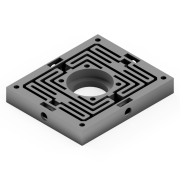
# Autodesk Inventor part: PinholeFlexMain
Saved by Autodesk Inventor 2022 (Build 260153000, 153)
## iProperties
Created: 2022-05-14
Part Number: PinholeFlexMain
Material: Acetal Resin, Black
Document SubType Name: Modeling
Designer: eganc
Density: 1.425 g/cm^3
Appearance: Smooth - Black
Author: eganc
Autodesk Inventor part; units mm, degrees
ref_plane "YZ Plane" through (0, 0, 0) normal (1, 0, 0) x (0, 1, 0)
ref_plane "XZ Plane" through (0, 0, 0) normal (0, 1, 0) x (-1, 0, 0)
ref_plane "XY Plane" through (0, 0, 0) normal (0, 0, 1) x (1, 0, 0)
sketch "Sketch1" plane through (0, 0, 0) normal (0, 1, 0) x (-1, 0, 0)
  line L0 (-14.5, 17.5) -> (14.5, 17.5)
  line L1 (14.5, 17.5) -> (14.5, -17.5)
  line L2 (14.5, -17.5) -> (-14.5, -17.5)
  line L3 (-14.5, -17.5) -> (-14.5, 17.5)
  line L4 (-14.5, 17.5) -> (14.5, -17.5) construction
  line L5 (14.5, 17.5) -> (-14.5, -17.5) construction
  point P0 (0, 0)
  dimension "d0" = 35
  dimension "d1" = 29
  constraints: 12 end point, 2 midpoint, 2 parallel, 1 horizontal, 1 perpendicular
  measures "d0" distance of L0.end L1.end
  measures "d1" distance of L1.end L2.end
extrude "Extrusion1" add sketch "Sketch1" along normal blind 5
sketch "Sketch2" plane through (0, 5, 0) normal (0, 1, 0) x (1, 0, 0)
  line L0 (12, -14.5) -> (-12, -14.5)
  line L1 (-12, -14.5) -> (-12, 14.5)
  line L2 (-12, 14.5) -> (12, 14.5)
  line L3 (12, 14.5) -> (12, -14.5)
  line L4 (12, -14.5) -> (-12, 14.5) construction
  line L5 (-12, -14.5) -> (12, 14.5) construction
  point P0 (0, 0)
  dimension "d4" = 24
  dimension "d5" = 29
  constraints: 12 end point, 2 midpoint, 2 parallel, 1 horizontal, 1 perpendicular
  measures "d4" distance of L1.end L2.end
  measures "d5" distance of L0.end L1.end
extrude "Extrusion2" cut sketch "Sketch2" against normal up to next
sketch "Sketch3" plane through (0, 5, 0) normal (0, 1, 0) x (1, 0, 0)
  line L0 (-14.5, -17.5) -> (14.5, -17.5) projected
  line L1 (0, -17.5) -> (0, 17.5) construction
  line L2 (14.5, 17.5) -> (-14.5, 17.5) projected
  line L3 (-14.5, 17.5) -> (-14.5, -17.5) projected
  line L4 (-14.5, 0) -> (14.5, 0) construction
  line L5 (14.5, -17.5) -> (14.5, 17.5) projected
  line L6 (12, -14.5) -> (-12, -14.5) projected
  line L7 (-2.3264, -14.5) -> (-2.3264, -13.6)
  line L8 (-2.3264, -13.6) -> (-11.1, -13.6)
  line L9 (-11.1, -13.6) -> (-11.1, -10.9)
  line L10 (-11.1, -10.9) -> (-2.3264, -10.9)
  line L11 (-2.3264, -10.9) -> (-2.3264, -10)
  line L12 (-2.3264, -10) -> (-11.1, -10)
  line L13 (-11.1, -10) -> (-11.1, -1.5)
  line L14 (-11.1, -1.5) -> (-8.4, -1.5)
  line L15 (-8.4, -1.5) -> (-8.4, -7.3)
  line L16 (-8.4, -7.3) -> (-2.3264, -7.3)
  line L17 (-2.3264, -7.3) -> (-2.3264, -6.43)
  line L18 (-2.3264, -6.43) -> (-7.5, -6.43)
  line L19 (-7.5, -6.43) -> (-7.5, -1)
  line L20 (-7.5, -1) -> (-8.25, -1)
  line L21 (-8.25, -1) -> (-8.25, 0)
  line L22 (-1.4, -14.5) -> (-1.4, -12.7)
  line L23 (-1.4, -12.7) -> (-10.2, -12.7)
  line L24 (-10.2, -12.7) -> (-10.2, -11.8)
  line L25 (-10.2, -11.8) -> (-1, -11.8)
  line L26 (-1, -11.8) -> (-1, -12.55)
  line L27 (-1, -12.55) -> (0, -12.55)
  line L28 (-9.3, -8.2) -> (-9.3, -2.4)
  line L29 (-9.3, -2.4) -> (-10.2, -2.4)
  line L30 (-10.2, -2.4) -> (-10.2, -9.1)
  line L31 (-10.2, -9.1) -> (0, -9.1)
  line L32 (-9.3, -8.2) -> (0, -8.2)
  line L33 (-2.3264, -14.5) -> (-1.4, -14.5)
  line L34 (-12, -14.5) -> (12, -14.5) projected
  line L35 (-2.3264, 14.5) -> (-2.3264, 13.6)
  line L36 (-2.3264, 13.6) -> (-11.1, 13.6)
  line L37 (-11.1, 13.6) -> (-11.1, 10.9)
  line L38 (-11.1, 10.9) -> (-2.3264, 10.9)
  line L39 (-2.3264, 10.9) -> (-2.3264, 10)
  line L40 (-2.3264, 10) -> (-11.1, 10)
  line L41 (-11.1, 10) -> (-11.1, 1.5)
  line L42 (-11.1, 1.5) -> (-8.4, 1.5)
  line L43 (-8.4, 1.5) -> (-8.4, 7.3)
  line L44 (-8.4, 7.3) -> (-2.3264, 7.3)
  line L45 (-2.3264, 7.3) -> (-2.3264, 6.43)
  line L46 (-2.3264, 6.43) -> (-7.5, 6.43)
  line L47 (-7.5, 6.43) -> (-7.5, 1)
  line L48 (-7.5, 1) -> (-8.25, 1)
  line L49 (-8.25, 1) -> (-8.25, 0)
  line L50 (-1.4, 14.5) -> (-1.4, 12.7)
  line L51 (-1.4, 12.7) -> (-10.2, 12.7)
  line L52 (-10.2, 12.7) -> (-10.2, 11.8)
  line L53 (-10.2, 11.8) -> (-1, 11.8)
  line L54 (-1, 11.8) -> (-1, 12.55)
  line L55 (-1, 12.55) -> (0, 12.55)
  line L56 (-9.3, 8.2) -> (-9.3, 2.4)
  line L57 (-9.3, 2.4) -> (-10.2, 2.4)
  line L58 (-10.2, 2.4) -> (-10.2, 9.1)
  line L59 (-10.2, 9.1) -> (0, 9.1)
  line L60 (-9.3, 8.2) -> (0, 8.2)
  line L61 (-2.3264, 14.5) -> (-1.4, 14.5)
  line L62 (2.3264, -14.5) -> (2.3264, -13.6)
  line L63 (2.3264, -13.6) -> (11.1, -13.6)
  line L64 (11.1, -13.6) -> (11.1, -10.9)
  line L65 (11.1, -10.9) -> (2.3264, -10.9)
  line L66 (2.3264, -10.9) -> (2.3264, -10)
  line L67 (2.3264, -10) -> (11.1, -10)
  line L68 (11.1, -10) -> (11.1, -1.5)
  line L69 (11.1, -1.5) -> (8.4, -1.5)
  line L70 (8.4, -1.5) -> (8.4, -7.3)
  line L71 (8.4, -7.3) -> (2.3264, -7.3)
  line L72 (2.3264, -7.3) -> (2.3264, -6.43)
  line L73 (2.3264, -6.43) -> (7.5, -6.43)
  line L74 (7.5, -6.43) -> (7.5, -1)
  line L75 (7.5, -1) -> (8.25, -1)
  line L76 (8.25, -1) -> (8.25, 0)
  line L77 (1.4, -14.5) -> (1.4, -12.7)
  line L78 (1.4, -12.7) -> (10.2, -12.7)
  line L79 (10.2, -12.7) -> (10.2, -11.8)
  line L80 (10.2, -11.8) -> (1, -11.8)
  line L81 (1, -11.8) -> (1, -12.55)
  line L82 (1, -12.55) -> (0, -12.55)
  line L83 (9.3, -8.2) -> (9.3, -2.4)
  line L84 (9.3, -2.4) -> (10.2, -2.4)
  line L85 (10.2, -2.4) -> (10.2, -9.1)
  line L86 (10.2, -9.1) -> (0, -9.1)
  line L87 (9.3, -8.2) -> (0, -8.2)
  line L88 (2.3264, -14.5) -> (1.4, -14.5)
  line L89 (2.3264, 6.43) -> (7.5, 6.43)
  line L90 (8.4, 7.3) -> (2.3264, 7.3)
  line L91 (9.3, 8.2) -> (0, 8.2)
  line L92 (10.2, 11.8) -> (1, 11.8)
  line L93 (10.2, 9.1) -> (0, 9.1)
  line L94 (1.4, 12.7) -> (10.2, 12.7)
  line L95 (10.2, 12.7) -> (10.2, 11.8)
  line L96 (2.3264, 13.6) -> (11.1, 13.6)
  line L97 (11.1, 10.9) -> (2.3264, 10.9)
  line L98 (2.3264, 10) -> (11.1, 10)
  line L99 (2.3264, 7.3) -> (2.3264, 6.43)
  line L100 (1, 11.8) -> (1, 12.55)
  line L101 (1, 12.55) -> (0, 12.55)
  line L102 (2.3264, 10.9) -> (2.3264, 10)
  line L103 (11.1, 13.6) -> (11.1, 10.9)
  line L104 (2.3264, 14.5) -> (2.3264, 13.6)
  line L105 (2.3264, 14.5) -> (1.4, 14.5)
  line L106 (1.4, 14.5) -> (1.4, 12.7)
  line L107 (11.1, 10) -> (11.1, 1.5)
  line L108 (11.1, 1.5) -> (8.4, 1.5)
  line L109 (8.4, 1.5) -> (8.4, 7.3)
  line L110 (9.3, 8.2) -> (9.3, 2.4)
  line L111 (7.5, 6.43) -> (7.5, 1)
  line L112 (7.5, 1) -> (8.25, 1)
  line L113 (8.25, 1) -> (8.25, 0)
  line L114 (9.3, 2.4) -> (10.2, 2.4)
  line L115 (10.2, 2.4) -> (10.2, 9.1)
  point P0 (0, 0)
  point P1 (-12, 14.5)
  point P2 (12, 14.5)
  dimension "d8" = 6.43
  dimension "d9" = 7.5
  dimension "d10" = 1.4
  dimension "d11" = 0.9
  dimension "d12" = 0.9
  dimension "d13" = 0.9
  dimension "d14" = 0.9
  dimension "d15" = 0.9
  dimension "d16" = 0.9
  dimension "d17" = 0.9
  dimension "d18" = 0.9
  dimension "d19" = 0.9
  dimension "d20" = 0.9
  dimension "d21" = 0.9
  dimension "d22" = 0.9
  dimension "d23" = 0.75
  dimension "d24" = 1
  dimension "d25" = 0.9
  dimension "d26" = 0.9
  dimension "d27" = 1.5
  dimension "d28" = 0.75
  dimension "d29" = 1
  constraints: 220 end point, 81 symmetric about line, 30 point on line, 19 perpendicular, 4 midpoint, 2 vertical, 1 collinear, 1 parallel
  measures "d8" distance between parallel lines of L4 L18
  measures "d9" distance between parallel lines of L1 L19
  measures "d10" distance between parallel lines of L1 L22
  measures "d11" distance between parallel lines of L8 L6
  measures "d12" distance between parallel lines of L23 L8
  measures "d13" distance between parallel lines of L25 L23
  measures "d14" distance between parallel lines of L10 L25
  measures "d15" distance between parallel lines of L12 L10
  measures "d16" distance between parallel lines of L31 L12
  measures "d17" distance between parallel lines of L32 L31
  measures "d18" distance between parallel lines of L16 L32
  measures "d19" distance between parallel lines of L19 L15
  measures "d20" distance between parallel lines of L28 L15
  measures "d21" distance between parallel lines of L30 L28
  measures "d22" distance between parallel lines of L13 L30
  measures "d23" distance of L25.end L26.end
  measures "d24" distance of L26.end L27.end
  measures "d25" distance between parallel lines of L14 L29
  measures "d26" distance between parallel lines of L24 L9
  measures "d27" distance between parallel lines of L4 L14
  measures "d28" distance between parallel lines of L19 L21
  measures "d29" distance between parallel lines of L4 L20
extrude "Extrusion3" add sketch "Sketch3" against normal up to surface (5 mm away) contours L6 L77 L78 L79 L80 L81 L82 L27 L26 L25 L24 L23 L22 L7 L8 L9 L10 L11 L12 L13 L14 L15 L16 L17 L18 L19 L20 L21 L49 L48 L47 L46 L45 L44 L43 L42 L41 L40 L39 L38 L37 L36 L35 L61 L50 L51 L52 L53 L54 L55 L101 L100 L92 L95 L94 L106 L105 L104 L96 L103 L97 L102 L98 L107 L108 L109 L90 L99 L89 L111 L112 L113 L76 L75 L74 L73 L72 L71 L70 L69 L68 L67 L66 L65 L64 L63 L62
sketch "Sketch4" plane through (0, 5, 0) normal (0, 1, 0) x (1, 0, 0)
  circle A0 centre (-11.5, -15.5) radius 1.25
  line L0 (-14.5, -17.5) -> (-9.5, -17.5)
  line L1 (-14.5, 17.5) -> (-14.5, -17.5)
  circle A1 centre (11.5, -15.5) radius 1.25
  circle A2 centre (11.5, 15.5) radius 1.25
  circle A3 centre (-11.5, 15.5) radius 1.25
  point P0 (0, 0)
  point P1 (0, 0)
  constraints: 4 centre point, 4 end point
sketch "Sketch5" plane through (0, 5, 0) normal (0, 1, 0) x (1, 0, 0)
  circle A0 centre (-12.5, -15.5) radius 0.8
  line L0 (-14.5, -17.5) -> (14.5, -17.5) projected
  line L1 (-14.5, 17.5) -> (-14.5, -17.5) projected
  line L2 (-12, -14.5) -> (-12, 14.5) projected
  line L3 (-11.1, -14.5) -> (-12, -14.5)
  line L4 (-12, -13.6) -> (-12, -14.5)
  line L5 (-12, 0) -> (12.1527, 0) construction
  line L6 (1.4, -14.5) -> (-1.4, -14.5) projected
  line L7 (0, -14.5) -> (0, 14.5) construction
  line L8 (-1.4, 14.5) -> (1.4, 14.5) projected
  circle A1 centre (-12.5, 15.5) radius 0.8
  circle A2 centre (12.5, -15.5) radius 0.8
  circle A3 centre (12.5, 15.5) radius 0.8
  point P0 (0, 0)
  dimension "d32" = 1.6
  dimension "d33" = 2
  dimension "d34" = 2
  dimension "d35" = 0.9
  constraints: 8 end point, 4 centre point, 3 midpoint, 3 symmetric about line, 2 horizontal, 1 collinear, 1 point on line, 3 other
  measures "d32" diameter of A0
  measures "d33" distance from line of L0 A0.centre
  measures "d34" distance from line of L1 A0.centre
  measures "d35" distance of L2.start L4.start
extrude "Extrusion4" cut sketch "Sketch5" against normal up to surface (5 mm away)
sketch "Sketch6" plane through (0, 5, 0) normal (0, 1, 0) x (1, 0, 0)
  line L0 (-14.5, 17.5) -> (-14.5, -17.5) projected
  line L1 (-14.5, 0) -> (14.5, 0) construction
  line L2 (14.5, -17.5) -> (14.5, 17.5) projected
  line L3 (-14.5, -17.5) -> (14.5, -17.5) projected
  line L4 (0, -17.5) -> (0, 17.5) construction
  line L5 (14.5, 17.5) -> (-14.5, 17.5) projected
  line L6 (-12, -14.5) -> (-2.3264, -14.5) projected
  line L7 (-11.1, -14.5) -> (-12, -13.6)
  line L8 (-12, -14.5) -> (-12, 14.5) projected
  line L9 (-11.1, -14.5) -> (-12, -14.5)
  line L10 (-12, -13.6) -> (-12, -14.5)
  line L11 (0, 17.5) -> (0, -17.5) construction
  line L12 (-11.1, 14.5) -> (-12, 13.6)
  line L13 (-11.1, 14.5) -> (-12, 14.5)
  line L14 (-12, 13.6) -> (-12, 14.5)
  line L15 (11.1, -14.5) -> (12, -13.6)
  line L16 (12, -14.5) -> (12, 14.5)
  line L17 (11.1, -14.5) -> (12, -14.5)
  line L18 (12, -13.6) -> (12, -14.5)
  line L19 (11.1, 14.5) -> (12, 13.6)
  line L20 (11.1, 14.5) -> (12, 14.5)
  line L21 (12, 13.6) -> (12, 14.5)
  point P0 (0, 0)
  dimension "d39" = 0.9
  dimension "d40" = 0.9
  constraints: 32 end point, 10 symmetric about line, 4 midpoint, 3 point on line, 2 collinear
  measures "d39" distance of L7.end L6.start
  measures "d40" distance of L7.start L6.start
extrude "Extrusion5" add sketch "Sketch6" against normal up to surface (5 mm away) contours L8 L7 L6 | L8 L13 L12 | L15 L16 L17 | L19 L20 L16
sketch "Sketch7" plane through (0, 5, 0) normal (0, 1, 0) x (1, 0, 0)
  line L0 (-7.25, -6.43) -> (-4, -6.43)
  line L1 (-7.5, -1.0473) -> (-7.5, -6.18)
  circle A0 centre (-6, -4.93) radius 0.8
  circle A1 centre (-6, 4.8353) radius 0.8
  circle A2 centre (6, 4.8353) radius 0.8
  circle A3 centre (6, -4.93) radius 0.8
  point P0 (0, 0)
  point P1 (0, 0)
  constraints: 4 centre point, 4 end point
extrude "Extrusion6" cut sketch "Sketch7" against normal up to surface (5 mm away)
fillet "Fillet1" radius 0.45 17 edges at (-1.4, 2.5, 12.7) (-10.2, 2.5, 12.7) (-11.1, 2.5, 10.9) (-10.2, 2.5, 9.1) (-8.4, 2.5, 7.3) (-2.3264, 2.5, 13.6) (-11.1, 2.5, 13.6) (-11.1, 2.5, 10) (-9.3, 2.5, 8.2) (-7.5, 2.5, 6.43) (-9.3, 2.5, 2.4) (-10.2, 2.5, 11.8) (-10.2, 2.5, 2.4) (-11.1, 2.5, 1.5) (-8.4, 2.5, 1.5) (-2.3264, 2.5, 10) (-2.3264, 2.5, 10.9)
mirror "Mirror1" about plane through (0, 0, 0) normal (0, 0, 1) of "Fillet1"
mirror "Mirror2" about plane through (0, 0, 0) normal (1, 0, 0) of "Fillet1", "Mirror1"
sketch "Sketch8" plane through (0, 5, 0) normal (0, 1, 0) x (1, 0, 0)
  circle A0 centre (0, 0) radius 5
  dimension "d47" = 10
  constraints: 1 centre point, 1 coincident
  measures "d47" diameter of A0
extrude "Extrusion7" cut sketch "Sketch8" against normal up to surface (5 mm away)
sketch "Sketch9" plane through (0, 5, 0) normal (0, 1, 0) x (1, 0, 0)
  circle A0 centre (0, 0) radius 6.45
  dimension "d50" = 12.9
  constraints: 1 centre point, 1 coincident
  measures "d50" diameter of A0
extrude "Extrusion8" cut sketch "Sketch9" against normal blind 3
sketch "Sketch10" plane through (0, 5, 0) normal (0, 1, 0) x (1, 0, 0)
  line L0 (-12.45, -2.5) -> (-14.05, -2.5)
  line L1 (-14.05, -2.5) -> (-14.05, 2.5)
  line L2 (-14.05, 2.5) -> (-12.45, 2.5)
  line L3 (-12.45, 2.5) -> (-12.45, -2.5)
  line L4 (-12.45, -2.5) -> (-14.05, 2.5) construction
  line L5 (-14.05, -2.5) -> (-12.45, 2.5) construction
  line L6 (-14.5, 17.5) -> (-14.5, -17.5) projected
  line L7 (-14.5, 0) -> (-12, 0) construction
  line L8 (-12, -13.6) -> (-12, 13.6) projected
  point P0 (0, 0)
  point P1 (-13.25, 0)
  point P2 (-13.25, 0)
  dimension "d53" = 1.6
  dimension "d54" = 5
  constraints: 14 end point, 6 midpoint, 2 parallel, 1 horizontal, 1 perpendicular
  measures "d53" distance of L1.end L2.end
  measures "d54" distance of L0.end L1.end
extrude "Extrusion9" cut sketch "Sketch10" against normal up to next
mirror "Mirror3" about plane through (0, 0, 0) normal (1, 0, 0) of "Extrusion9"
sketch "Sketch11" plane through (0, 5, 0) normal (0, 1, 0) x (1, 0, 0)
  line L0 (2.5, -16.8) -> (-2.5, -16.8)
  line L1 (-2.5, -16.8) -> (-2.5, -15.2)
  line L2 (-2.5, -15.2) -> (2.5, -15.2)
  line L3 (2.5, -15.2) -> (2.5, -16.8)
  line L4 (2.5, -16.8) -> (-2.5, -15.2) construction
  line L5 (-2.5, -16.8) -> (2.5, -15.2) construction
  line L6 (-14.5, -17.5) -> (14.5, -17.5) projected
  line L7 (-1.4, -14.5) -> (1.4, -14.5) projected
  line L8 (0, -14.5) -> (0, -17.5) construction
  point P0 (0, 0)
  point P1 (0, -16)
  point P2 (0, -16)
  dimension "d57" = 1.6
  dimension "d58" = 5
  dimension "d59" = 0.7
  constraints: 14 end point, 6 midpoint, 2 parallel, 1 horizontal, 1 perpendicular
  measures "d57" distance of L0.end L1.end
  measures "d58" distance of L0.start L0.end
  measures "d59" distance between parallel lines of L6 L0
extrude "Extrusion10" cut sketch "Sketch11" against normal up to next
mirror "Mirror4" about plane through (0, 0, 0) normal (0, 0, 1) of "Extrusion10"
sketch "Sketch12" plane through (14.5, 0, -17.5) normal (0, 0, -1) x (-1, 0, 0)
  line L0 (14.5, 0) -> (14.5, 5) construction
  line L1 (23.35, 5) -> (5.65, 5) projected
  circle A0 centre (14.5, 2.5) radius 1.3
  dimension "d62" = 2.6
  constraints: 2 end point, 2 midpoint, 1 centre point
  measures "d62" diameter of A0
extrude "Extrusion11" cut sketch "Sketch12" against normal up to surface (3 mm away)
mirror "Mirror5" about plane through (0, 0, 0) normal (0, 0, 1) of "Extrusion11"
sketch "Sketch13" plane through (14.5, 0, 17.5) normal (1, 0, 0) x (0, 0, -1)
  line L0 (18.5, 5) -> (16.5, 5) projected
  line L1 (17.5, 5) -> (17.5, 0) construction
  circle A0 centre (17.5, 2.5) radius 1.3
  dimension "d65" = 2.6
  constraints: 2 end point, 2 midpoint, 1 centre point, 1 vertical
  measures "d65" diameter of A0
extrude "Extrusion12" cut sketch "Sketch13" against normal up to surface (2.5 mm away)
mirror "Mirror6" about plane through (0, 0, 0) normal (1, 0, 0) of "Extrusion12"
sketch "Sketch14" plane through (0, 5, 0) normal (0, 1, 0) x (1, 0, 0)
  circle A0 centre (-12.5, -15.5) radius 0.8 projected
  circle A1 centre (12.5, -15.5) radius 0.8 projected
  circle A2 centre (-12.5, 15.5) radius 0.8 projected
  circle A3 centre (12.5, 15.5) radius 0.8 projected
  circle A4 centre (0, 0) radius 6.45 projected
  circle A5 centre (0, 0) radius 5 projected
  line L0 (14.5, -17.5) -> (14.5, 17.5) projected
  line L1 (14.5, 17.5) -> (-14.5, 17.5) projected
  line L2 (-14.5, 17.5) -> (-14.5, -17.5) projected
  line L3 (-14.5, -17.5) -> (14.5, -17.5) projected
equation "\"d11\" = SW"
equation "\"d12\" = SW"
equation "\"d13\" = SW"
equation "\"d14\" = SW"
equation "\"d15\" = SW"
equation "\"d16\" = SW"
equation "\"d17\" = SW"
equation "\"d18\" = SW"
equation "\"d19\" = SW"
equation "\"d20\" = SW"
equation "\"d21\" = SW"
equation "\"d22\" = SW"
equation "\"d25\" = SW"
equation "\"d26\" = SW"
equation "\"d35\" = SW"
equation "\"d39\" = SW"
equation "\"d40\" = SW"
equation "\"d46\" = 0.5 * SW"
equation "\"SW\" = 0.9"
body "Solid1"
